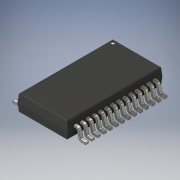
# Autodesk Inventor part: Semiconductor_TSSOP-28
Saved by Autodesk Inventor 2018 (Build 220112000, 112)
## iProperties
Created: 2016-07-22
Part Number: Semiconductor_TSSOP-28
Material: ABS Plastic
Document SubType Name: Modeling
Designer: Bradley
Density: 1.06 g/cm^3
Appearance: Smooth - Black
Mass: 0.00993513 g
Surface Area: 0.40182 cm^2
Volume: 0.00937276 cm^3
Author: Bradley
Autodesk Inventor part; units mm, degrees
ref_plane "YZ Plane" through (0, 0, 0) normal (1, 0, 0) x (0, 1, 0)
ref_plane "XZ Plane" through (0, 0, 0) normal (0, 1, 0) x (-1, 0, 0)
ref_plane "XY Plane" through (0, 0, 0) normal (0, 0, 1) x (1, 0, 0)
sketch "Sketch1" plane through (0, 0, 0) normal (0, 1, 0) x (-1, 0, 0)
  line L0 (-2.65, 5.1) -> (2.65, 5.1)
  line L1 (2.65, 5.1) -> (2.65, -5.1)
  line L2 (2.65, -5.1) -> (-2.65, -5.1)
  line L3 (-2.65, -5.1) -> (-2.65, 5.1)
  line L4 (-2.65, 5.1) -> (2.65, -5.1) construction
  line L5 (2.65, 5.1) -> (-2.65, -5.1) construction
  point P0 (0, 0)
  dimension "d0" = 5.3
  dimension "d1" = 10.2
  constraints: 12 end point, 2 midpoint, 2 parallel, 1 horizontal, 1 perpendicular
  measures "d0" distance of L1.end L2.end
  measures "d1" distance of L0.end L1.end
extrude "Extrusion1" add sketch "Sketch1" along normal blind 0.9 draft -5
sketch "Sketch2" plane through (0, 0, 0) normal (0, -1, 0) x (1, 0, 0)
  line L0 (2.65, 5.1) -> (-2.65, 5.1) projected
  line L1 (2.65, 5.1) -> (-2.65, 5.1) projected
  line L2 (-2.65, 5.1) -> (-2.65, -5.1) projected
  line L3 (-2.65, -5.1) -> (2.65, -5.1) projected
  line L4 (2.65, -5.1) -> (2.65, 5.1) projected
  point P0 (0, 0)
extrude "Extrusion2" add sketch "Sketch2" along normal blind 0.9 draft -5
fillet "Fillet1" radius 0.1 8 edges at (-2.5713, 0.9, 0) (0, 0.9, 5.0213) (0, 0.9, -5.0213) (2.5713, 0.9, 0) (2.5713, -0.9, 0) (0, -0.9, 5.0213) (-2.5713, -0.9, 0) (0, -0.9, -5.0213)
sketch "Sketch3" plane through (0, 0, 0) normal (0, 1, 0) x (-1, 0, 0)
  line L0 (2.65, 5.1) -> (2.65, -5.1) projected
  line L1 (-2.65, 5.1) -> (2.65, 5.1) projected
  line L2 (2.65, 4.375) -> (2.85, 4.375)
  line L3 (2.85, 4.375) -> (2.85, 4.075)
  line L4 (2.85, 4.075) -> (2.65, 4.075)
  line L5 (2.65, 4.075) -> (2.65, 4.375)
  line L6 (-2.65, -5.1) -> (-2.65, 5.1) projected
  line L7 (-2.65, 4.375) -> (-2.85, 4.375)
  line L8 (-2.85, 4.375) -> (-2.85, 4.075)
  line L9 (-2.85, 4.075) -> (-2.65, 4.075)
  line L10 (-2.65, 4.075) -> (-2.65, 4.375)
  line L11 (-2.65, 4.075) -> (2.65, 4.075)
  line L12 (2.65, 4.075) -> (2.65, 4.375)
  line L13 (2.65, 4.375) -> (-2.65, 4.375)
  line L14 (-2.65, 4.375) -> (-2.65, 4.075)
  point P0 (0, 0)
  point P1 (2.65, 4.225)
  dimension "d7" = 0.3
  dimension "d8" = 4.225
  dimension "d9" = 0.2
  constraints: 24 end point, 6 parallel, 4 point on line, 3 horizontal, 3 perpendicular, 1 collinear, 1 midpoint
  measures "d7" distance of L2.end L3.end
  measures "d8" vertical distance of point (2.65, 4.225) point (0, 0)
  measures "d9" distance of L3.end L4.end
extrude "Extrusion3" add sketch "Sketch3" along normal blind 0.2 contours L2 L3 L4 L0 | L0 L11 L6 L13 | L6 L9 L8 L7
sketch "Sketch4" plane through (-2.85, 0, 4.375) normal (0, 0, 1) x (1, 0, 0)
  line L0 (0.2175, 0.2) -> (0.2, 0) projected
  line L1 (0, 0.2) -> (0.2175, 0.2) projected
  line L2 (0, 0) -> (0, 0.2) projected
  line L3 (0, 0) -> (0.2, 0) projected
  line L4 (5.5, 0) -> (5.4825, 0.2) projected
  line L5 (5.5, 0) -> (5.7, 0) projected
  line L6 (5.7, 0) -> (5.7, 0.2) projected
  line L7 (5.4825, 0.2) -> (5.7, 0.2) projected
  line L8 (0, 0) -> (0.2, 0) projected
  arc A0 (0, 0) -> (-0.1456, -0.1138) centre (0, -0.15) ccw
  arc A1 (-0.6396, -1) -> (-0.3, -0.7345) centre (-0.6396, -0.65) ccw
  line L9 (0, 0.2) -> (0.2175, 0.2) projected
  arc A2 (0, 0.2) -> (-0.3396, -0.0655) centre (0, -0.15) ccw
  arc A3 (-0.6396, -0.8) -> (-0.4941, -0.6862) centre (-0.6396, -0.65) ccw
  line L10 (-0.6396, -1) -> (-1.05, -1)
  line L11 (-1.05, -1) -> (-1.05, -0.8)
  line L12 (-1.05, -0.8) -> (-0.6396, -0.8)
  line L13 (-0.3396, -0.0655) -> (-0.4941, -0.6862)
  line L14 (-0.1456, -0.1138) -> (-0.3, -0.7345)
  line L15 (5.3296, -0.9) -> (0.3704, -0.9) projected
  line L16 (0, 0.2) -> (0, 0)
  line L17 (0.3704, 0.9) -> (5.3296, 0.9) projected
  line L18 (2.85, 0.5) -> (2.85, -0.5)
  line L19 (5.7, 0) -> (5.7, 0.2)
  arc A4 (5.8456, -0.1138) -> (5.7, 0) centre (5.7, -0.15) ccw
  arc A5 (6, -0.7345) -> (6.3396, -1) centre (6.3396, -0.65) ccw
  arc A6 (6.0396, -0.0655) -> (5.7, 0.2) centre (5.7, -0.15) ccw
  arc A7 (6.1941, -0.6862) -> (6.3396, -0.8) centre (6.3396, -0.65) ccw
  line L20 (6.3396, -1) -> (6.75, -1)
  line L21 (6.75, -1) -> (6.75, -0.8)
  line L22 (6.75, -0.8) -> (6.3396, -0.8)
  line L23 (6.0396, -0.0655) -> (6.1941, -0.6862)
  line L24 (5.8456, -0.1138) -> (6, -0.7345)
  point P0 (2.85, 0)
  dimension "d12" = 0.15
  dimension "d13" = 0.15
  dimension "d16" = 0.75
  dimension "d25" = 7.8
  dimension "d30" = 0.1
  constraints: 26 end point, 16 point on circle, 12 symmetric about line, 8 centre point, 6 tangent, 4 coincident, 2 equal length, 2 perpendicular, 1 horizontal, 1 parallel, 4 other
  measures "d12" radius of A0
  measures "d13" radius of A3
  measures "d16" distance from line of L11 L14.end
  measures "d25" distance between parallel lines of L21 L11
  measures "d30" distance between parallel lines of L10 L15
extrude "Extrusion4" add sketch "Sketch4" against normal up to surface (0.3 mm away) contours L2 A0 L14 A1 L10 L11 L12 A3 L13 A2 | L6 A6 L23 A7 L22 L21 L20 A5 L24 A4
pattern_linear "Rectangular Pattern1" count 14 spacing 0.65 along (0, 0, -1) of "Extrusion4", "Extrusion3"
sketch "Sketch5" plane through (0, 0.9, 0) normal (0, 1, 0) x (1, 0, 0)
  line L0 (2.4796, -4.9296) -> (-2.4796, -4.9296) projected
  line L1 (2.4796, 4.9296) -> (2.4796, -4.9296) projected
  line L2 (-2.4796, 4.9296) -> (2.4796, 4.9296) projected
  line L3 (-2.4796, -4.9296) -> (-2.4796, 4.9296) projected
  circle A0 centre (-2.15, 4.6) radius 0.15
  circle A1 centre (-2.15, 4.6) radius 0.3296 construction
  line L4 (-2.4796, -4.9296) -> (-2.4796, 4.9296) projected
  line L5 (-2.4796, -4.9296) -> (2.4796, -4.9296) construction
  line L6 (-2.4796, 4.9296) -> (2.4796, 4.9296) construction
  line L7 (-2.65, 5.1) -> (2.65, 5.1) projected
  point P0 (0, 0)
  dimension "d26" = 0.5
  dimension "d27" = 0.3
  constraints: 2 centre point, 2 tangent, 1 coincident
  measures "d26" distance from line of A0.centre L7
  measures "d27" diameter of A0
extrude "Extrusion5" add sketch "Sketch5" along normal blind 0.01 and the other way blind 0.255 contours A0
equation "\"d13\" = d12"
body "Solid1"
